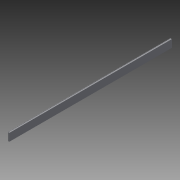
# Autodesk Inventor part: Mirroir
Saved by Autodesk Inventor 2015 SP1 (Build 190203100, 203)
## iProperties
Created: 2015-03-28
Part Number: Mirroir
Material: Generic
Document SubType Name: Modeling
Designer: Cyril
Density: 1 g/cm^3
Appearance: Default
Author: Cyril
Autodesk Inventor part; units mm, degrees
ref_plane "YZ Plane" through (0, 0, 0) normal (1, 0, 0) x (0, 1, 0)
ref_plane "XZ Plane" through (0, 0, 0) normal (0, 1, 0) x (-1, 0, 0)
ref_plane "XY Plane" through (0, 0, 0) normal (0, 0, 1) x (1, 0, 0)
sketch "Sketch1" plane through (0, 0, 0) normal (0, 0, 1) x (1, 0, 0)
  line L0 (-8, -50) -> (8, -50) construction
  line L1 (8, -50) -> (8, 50) construction
  line L2 (8, 50) -> (-8, 50) construction
  line L3 (-8, 50) -> (-8, -50)
  line L4 (-8, -50) -> (8, 50) construction
  line L5 (8, -50) -> (-8, 50) construction
  line L6 (-8, -50) -> (-6, -50)
  line L7 (-6, -47) -> (8, -44)
  line L8 (-6, -47) -> (-6, -50)
  line L9 (8, -44) -> (8, 44)
  line L10 (8, 44) -> (-6, 47)
  line L11 (-6, 47) -> (-6, 50)
  line L12 (-6, 50) -> (-8, 50)
  line L13 (-8, 0) -> (8, 0) construction
  point P0 (0, 0)
  dimension "d0" = 100
  dimension "d1" = 16
  dimension "d4" = 3
  dimension "d5" = 3
  dimension "d6" = 2
  dimension "d7" = 6
  constraints: 26 end point, 6 point on line, 4 midpoint, 2 horizontal, 2 parallel, 1 perpendicular, 5 other
  measures "d0" distance of L2.end L0.start
  measures "d1" distance of L1.end L2.end
  measures "d4" distance of L7.start L6.end
  measures "d5" distance of L10.end L11.end
  measures "d6" distance of L0.start L6.end
  measures "d7" distance from line of L7.end L0
extrude "Extrusion1" add sketch "Sketch1" along normal mid plane 2000
body "Solid1"
